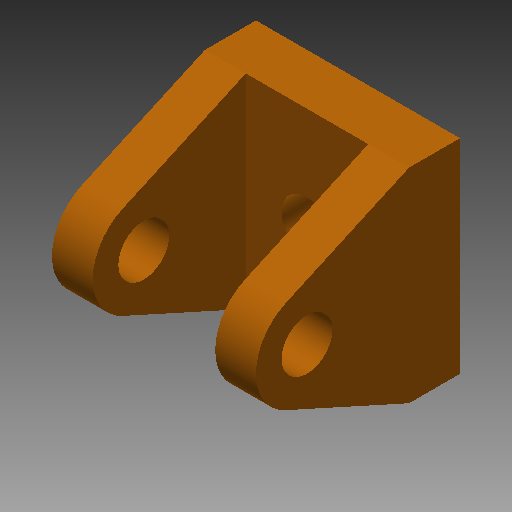
# Autodesk Inventor part: Joint
Saved by Autodesk Inventor 2017 (Build 210142000, 142)
## iProperties
Created: 2014-03-04
Part Number: Joint
Material: Aluminum 6061
Document SubType Name: Modeling
Designer: John
Density: 2.71 g/cm^3
Appearance: Orange
Mass: 18.3367 g
Surface Area: 35.6297 cm^2
Volume: 6.76632 cm^3
Author: John
Autodesk Inventor part; units mm, degrees
ref_plane "YZ Plane" through (0, 0, 0) normal (1, 0, 0) x (0, 1, 0)
ref_plane "XZ Plane" through (0, 0, 0) normal (0, 1, 0) x (-1, 0, 0)
ref_plane "XY Plane" through (0, 0, 0) normal (0, 0, 1) x (1, 0, 0)
sketch "Sketch1" plane through (0, 0, 0) normal (0, 0, 1) x (1, 0, 0)
  line L0 (0, 0) -> (25.4, 0)
  line L1 (25.4, 0) -> (25.4, 25.4)
  line L2 (25.4, 25.4) -> (0, 25.4)
  line L3 (0, 25.4) -> (0, 0)
  dimension "d0" = 25.4
  dimension "d1" = 25.4
  constraints: 8 end point, 2 parallel, 1 horizontal, 1 perpendicular
  measures "d0" distance of L2.end L1.end
  measures "d1" distance of L1.end L0.end
extrude "Extrusion1" add sketch "Sketch1" along normal blind 25.4
sketch "Sketch2" plane through (25.4, 0, 0) normal (1, 0, 0) x (0, 0, -1)
  line L0 (0, 0) -> (0, 25.4) projected
  line L1 (0, 25.4) -> (-25.4, 25.4) projected
  line L2 (-25.4, 0) -> (-25.4, 25.4) projected
  line L3 (0, 0) -> (-25.4, 0) projected
  circle A0 centre (-19.05, 12.7) radius 6.35
  line L4 (-21.6626, 18.4876) -> (-6.35, 25.4)
  line L5 (-21.6626, 6.9124) -> (-6.35, 0)
  line L6 (0, 12.7) -> (-19.05, 12.7) construction
  dimension "d4" = 12.7
  dimension "d5" = 6.35
  constraints: 6 end point, 3 tangent, 2 point on circle, 2 point on line, 1 centre point, 1 midpoint, 1 parallel, 1 other
  measures "d4" diameter of A0
  measures "d5" distance from line of L0 L5.end
extrude "Extrusion2" cut sketch "Sketch2" against normal through all contours L3 L2 A0 L5 | L4 A0 L2 L1
sketch "Sketch3" plane through (25.4, 0, 0) normal (1, 0, 0) x (0, 0, -1)
  arc A0 (-21.6626, 18.4876) -> (-21.6626, 6.9124) centre (-19.05, 12.7) ccw projected
hole "Hole1" at (25.4, 12.7, 19.05) direction (-1, 0, 0) diameter 6.35 end through all
sketch "Sketch4" plane through (0, 25.4, 0) normal (0, 1, 0) x (1, 0, 0)
  line L0 (0, -6.35) -> (25.4, -6.35) projected
  line L1 (25.4, 0) -> (25.4, -6.35) projected
  line L2 (0, 0) -> (0, -6.35) projected
  line L3 (25.4, -25.4) -> (0, -25.4) projected
  line L4 (5.08, -6.35) -> (20.32, -6.35)
  line L5 (20.32, -6.35) -> (20.32, -25.4)
  line L6 (20.32, -25.4) -> (5.08, -25.4)
  line L7 (5.08, -25.4) -> (5.08, -6.35)
  dimension "d15" = 5.08
  dimension "d16" = 5.08
  constraints: 8 end point, 2 parallel, 2 point on line, 1 horizontal, 1 perpendicular
  measures "d15" distance between parallel lines of L1 L5
  measures "d16" distance between parallel lines of L2 L7
extrude "Extrusion3" cut sketch "Sketch4" against normal through all
sketch "Sketch5" plane through (0, 0, 0) normal (0, 0, -1) x (-1, 0, 0)
  line L0 (-25.4, 25.4) -> (0, 0) construction
  circle A0 centre (-12.7, 12.7) radius 3.175
  dimension "d19" = 6.35
  constraints: 2 end point, 1 centre point, 1 midpoint
  measures "d19" diameter of A0
extrude "Extrusion4" cut sketch "Sketch5" against normal through all
equation "\"d16\" = d15"
body "Solid1"
